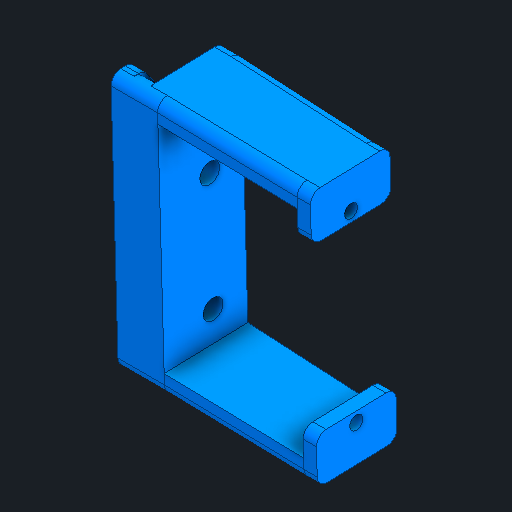
# Autodesk Inventor part: servo_mount
Saved by Autodesk Inventor 2023 (Build 270158030, 158C)
## iProperties
Created: 2022-03-29
Part Number: servo_mount
Material: Generic
Document SubType Name: Modeling
Designer: kardo
Density: 1 g/cm^3
Appearance: Blue Plastic
Author: kardo
Autodesk Inventor part; units mm, degrees
ref_plane "YZ Plane" through (0, 0, 0) normal (1, 0, 0) x (0, 1, 0)
ref_plane "XZ Plane" through (0, 0, 0) normal (0, 1, 0) x (-1, 0, 0)
ref_plane "XY Plane" through (0, 0, 0) normal (0, 0, 1) x (1, 0, 0)
derived "stencil_frame.ipt"
sketch "sk_servo_mount" plane through (-54.6, 0, 0) normal (1, 0, 0) x (0, 1, 0)
  line L0 (-254.1001, 21.0191) -> (9.48, 28.5282) construction
  line L1 (-363, 4666.1952) -> (-363, -2045.0469) construction
  line L2 (0, 4666.1952) -> (0, -2045.0469) construction
  line L3 (-204.8284, 22.4228) -> (-205.0163, 29.0201) construction
  line L4 (-205.0163, 29.0201) -> (-187.0237, 29.5327) construction
  line L5 (-187.0237, 29.5327) -> (-186.8357, 22.9354) construction
  point P0 (0, 0)
  point P1 (-196.02, 29.2764)
ref_plane "plane_cowl_left" through (-54.6, 0, 0) normal (1, 0, 0) x (0, 1, 0)
derived "parameters_frame.ipt"
derived "parameters_powertrain.ipt"
derived "parameters_hardware.ipt"
ref_plane "plane_inner_stringer" through (-54.6, -254.1001, 21.0191) normal (1, 0, 0) x (0, 0.9995944, 0.0284775)
ref_plane "plane_fastening" through (-28.6, -254.1001, 21.0191) normal (1, 0, 0) x (0, 0.9995944, 0.0284775)
ref_plane "plane_servo_rod_joint" through (-14.6, -254.1001, 21.0191) normal (1, 0, 0) x (0, 0.9995944, 0.0284775)
sketch "sk_fastening" plane through (-28.6, -254.1001, 21.0191) normal (1, 0, 0) x (0, 0.9995944, 0.0284775)
  line L0 (49.2917, 6.6) -> (67.2917, 6.6) construction
  line L1 (58.2917, 6.6) -> (58.2917, 106.6) construction
  line L2 (58.2917, 106.6) -> (158.2917, 106.6) construction
  line L3 (158.2917, 106.6) -> (158.2917, 22.6) construction
  line L4 (158.2917, 22.6) -> (66.2917, 22.6) construction
  line L5 (66.2917, 22.6) -> (66.2917, 8.6) construction
  line L6 (66.2917, 8.6) -> (61.2917, 8.6) construction
  line L7 (44.7917, 14.6) -> (44.7917, 2.6)
  line L8 (44.7917, 2.6) -> (48.7917, 2.6)
  line L9 (48.7917, 2.6) -> (48.7917, 14.6)
  line L10 (48.7917, 14.6) -> (44.7917, 14.6)
  line L11 (73.7917, 14.6) -> (73.7917, 2.6)
  line L12 (73.7917, 2.6) -> (77.7917, 2.6)
  line L13 (77.7917, 2.6) -> (77.7917, 14.6)
  line L14 (77.7917, 14.6) -> (73.7917, 14.6)
  line L15 (48.7917, 14.6) -> (73.7917, 14.6) construction
  line L16 (73.7917, 2.6) -> (48.7917, 2.6) construction
  line L17 (61.2917, 2.6) -> (61.2917, 14.6) construction
  line L18 (44.7917, 14.6) -> (41.7917, 14.6)
  line L19 (41.7917, 14.6) -> (41.7917, 2.6)
  line L20 (41.7917, 2.6) -> (44.7917, 2.6)
  line L21 (77.7917, 14.6) -> (80.7917, 14.6)
  line L22 (80.7917, 14.6) -> (80.7917, 2.6)
  line L23 (80.7917, 2.6) -> (77.7917, 2.6)
  line L24 (47.2917, 8.6) -> (48.7917, 8.6) construction
  line L25 (73.7917, 8.6) -> (75.2917, 8.6) construction
  point P0 (253.3985, -28.2467)
  point P1 (61.2917, 8.6)
  dimension "d46" = 100
  dimension "d47" = 84
  dimension "d49" = 100
  dimension "d50" = 92
  dimension "d52" = 14
  dimension "d53" = 5
  dimension "d54" = 25
  dimension "d55" = 33
  dimension "d56" = 3
  dimension "d57" = 3
  dimension "d58" = 12
  dimension "d59" = 28
  constraints: 50 end point, 8 collinear, 8 perpendicular, 7 parallel, 5 midpoint, 2 point on line, 1 coincident, 1 other
  measures "d46" distance of L1.end L2.end
  measures "d47" distance of L2.end L3.end
  measures "d49" distance of L1.start L1.end
  measures "d50" distance of L3.end L4.end
  measures "d52" distance of L4.end L5.end
  measures "d53" distance of L6.end L5.end
  measures "d54" distance between parallel lines of L11 L9
  measures "d55" distance between parallel lines of L13 L7
  measures "d56" distance of L7.start L18.end
  measures "d57" distance of L13.end L21.end
  measures "d58" distance of L21.end L22.end
  measures "d59" distance of L25.end L24.start
sketch "sk_base" plane through (-54.6, -254.1001, 21.0191) normal (1, 0, 0) x (0, 0.9995944, 0.0284775)
  line L0 (44.7917, 14.6) -> (41.7917, 14.6) construction
  line L1 (41.7917, 14.6) -> (41.7917, 2.6) construction
  line L2 (41.7917, 2.6) -> (44.7917, 2.6) construction
  line L3 (80.7917, 2.6) -> (77.7917, 2.6) construction
  line L4 (80.7917, 14.6) -> (80.7917, 2.6) construction
  line L5 (77.7917, 14.6) -> (80.7917, 14.6) construction
  line L6 (49.2917, 6.6) -> (67.2917, 6.6) construction
  line L7 (0, 0) -> (263.6871, 0) construction
  line L8 (41.7917, 1.5) -> (80.7917, 1.5)
  line L9 (80.7917, 1.5) -> (80.7917, 14.1)
  line L10 (80.7917, 14.1) -> (41.7917, 14.1)
  line L11 (41.7917, 14.1) -> (41.7917, 1.5)
  line L12 (49.2917, 6.6) -> (41.7917, 6.6) construction
  line L13 (49.2917, 6.6) -> (49.2917, 14.1) construction
  line L14 (67.2917, 6.6) -> (80.7917, 6.6) construction
  line L15 (67.2917, 6.6) -> (67.2917, 14.1) construction
  point P0 (253.3985, -28.2467)
  point P1 (61.2917, 8.6)
  point P2 (58.2917, 6.6)
  dimension "d60" = 22.5
  dimension "d61" = 16.5
  dimension "d62" = 18
  dimension "d64" = 1.5
  dimension "d65" = 7.5
  dimension "d66" = 16.5
  dimension "d67" = 22.5
  constraints: 16 end point, 6 perpendicular, 4 point on line, 2 parallel
  measures "d60" distance from line of L4 point (58.292, 6.6)
  measures "d61" distance from line of L1 point (58.292, 6.6)
  measures "d62" distance of L6.start L6.end
  measures "d64" distance between parallel lines of L7 L8
  measures "d65" distance of L12.start L13.end
  measures "d66" distance from line of point (58.292, 6.6) L11
  measures "d67" distance from line of point (58.292, 6.6) L9
ref_plane "plane_column_bottom" through (-52.1, -254.1001, 21.0191) normal (1, 0, 0) x (0, 0.9995944, 0.0284775)
ref_plane "plane_outer_plate" through (-57.1, -254.1001, 21.0191) normal (1, 0, 0) x (0, 0.9995944, 0.0284775)
sketch "sk_hex_holes" plane through (-57.1, -254.1001, 21.0191) normal (1, 0, 0) x (0, 0.9995944, 0.0284775)
  line L0 (50.8794, 9.35) -> (52.4671, 6.6)
  line L1 (52.4671, 6.6) -> (50.8794, 3.85)
  line L2 (50.8794, 3.85) -> (47.704, 3.85)
  line L3 (47.704, 3.85) -> (46.1163, 6.6)
  line L4 (46.1163, 6.6) -> (47.704, 9.35)
  line L5 (47.704, 9.35) -> (50.8794, 9.35)
  line L6 (68.8794, 9.35) -> (70.4671, 6.6)
  line L7 (70.4671, 6.6) -> (68.8794, 3.85)
  line L8 (68.8794, 3.85) -> (65.704, 3.85)
  line L9 (65.704, 3.85) -> (64.1163, 6.6)
  line L10 (64.1163, 6.6) -> (65.704, 9.35)
  line L11 (65.704, 9.35) -> (68.8794, 9.35)
  point P0 (253.3985, -28.2467)
  point P1 (49.2917, 6.6)
  point P2 (67.2917, 6.6)
  point P3 (49.2917, 6.6)
  point P4 (67.2917, 6.6)
  dimension "d102" = 5.5
  constraints: 24 end point, 2 coincident, 2 collinear, 26 other
  measures "d102" distance between parallel lines of L2 L5
sketch "sk_bridge" plane through (-54.6, -254.1001, 21.0191) normal (1, 0, 0) x (0, 0.9995944, 0.0284775)
  line L0 (80.7917, 14.1) -> (41.7917, 14.1) projected
  line L1 (41.7917, 14.1) -> (41.7917, 1.5) projected
  line L2 (80.7917, 1.5) -> (80.7917, 14.1) projected
  line L3 (41.7917, 11.1) -> (80.7917, 11.1)
  point P0 (253.3985, -28.2467)
  dimension "d70" = 3
  constraints: 2 end point, 2 point on line, 1 parallel
  measures "d70" distance between parallel lines of L0 L3
sketch "sk_backplate" plane through (-57.1, -254.1001, 21.0191) normal (1, 0, 0) x (0, 0.9995944, 0.0284775)
  line L0 (41.7917, 14.1) -> (41.7917, 1.5) construction
  line L1 (80.7917, 14.1) -> (41.7917, 14.1) projected
  line L2 (80.7917, 1.5) -> (80.7917, 14.1) construction
  line L3 (68.8794, 3.85) -> (65.704, 3.85) projected
  line L4 (50.8794, 3.85) -> (47.704, 3.85) projected
  line L5 (80.7917, 14.1) -> (80.7917, 11.1)
  line L6 (72.0548, 3.85) -> (68.8794, 3.85)
  line L7 (65.704, 3.85) -> (50.8794, 3.85)
  line L8 (47.704, 3.85) -> (44.5286, 3.85)
  line L9 (41.7917, 14.1) -> (41.7917, 11.1)
  line L10 (47.704, 3.85) -> (46.1163, 6.6) construction
  line L11 (41.7917, 11.1) -> (80.7917, 11.1) construction
  line L12 (70.4671, 6.6) -> (68.8794, 3.85) construction
  line L13 (44.5286, 3.85) -> (42.9408, 6.6)
  line L14 (42.9408, 6.6) -> (41.7917, 11.1)
  line L15 (80.7917, 11.1) -> (73.6426, 6.6)
  line L16 (73.6426, 6.6) -> (72.0548, 3.85)
  point P0 (253.3985, -28.2467)
  constraints: 18 end point, 4 equal length, 2 collinear, 2 parallel
ref_plane "plane_column_top" through (-30.6, -254.1001, 21.0191) normal (1, 0, 0) x (0, 0.9995944, 0.0284775)
extrude "extrude_fastening_plates" add sketch "sk_fastening" against normal up to surface (2 mm away)
extrude "extrude_backplate" add sketch "sk_backplate" against normal blind 2
extrude "extrude_front_plate" add sketch "sk_base" along normal up to surface (2.5 mm away)
extrude "extrude_bridge" add sketch "sk_bridge" against normal up to surface (2.5 mm away)
sketch "sk_column_bottom_1" plane through (-52.1, -254.1001, 21.0191) normal (1, 0, 0) x (0, 0.9995944, 0.0284775)
  line L0 (80.7917, 14.1) -> (41.7917, 14.1) construction
  line L1 (41.7917, 1.5) -> (80.7917, 1.5) construction
  line L2 (44.7917, 14.6) -> (44.7917, 2.6) construction
  line L3 (41.7917, 14.6) -> (41.7917, 2.6) construction
  line L4 (41.7917, 14.1) -> (44.7917, 14.1)
  line L5 (44.7917, 14.1) -> (44.7917, 1.5)
  line L6 (44.7917, 1.5) -> (41.7917, 1.5)
  line L7 (41.7917, 1.5) -> (41.7917, 14.1)
  point P0 (253.3985, -28.2467)
  constraints: 8 end point, 4 collinear
sketch "sk_column_top_1" plane through (-30.6, -254.1001, 21.0191) normal (1, 0, 0) x (0, 0.9995944, 0.0284775)
  line L0 (41.7917, 14.6) -> (41.7917, 2.6) projected
  line L1 (44.7917, 14.6) -> (41.7917, 14.6) projected
  line L2 (44.7917, 14.6) -> (44.7917, 2.6) projected
  line L3 (41.7917, 2.6) -> (44.7917, 2.6) projected
  point P0 (253.3985, -28.2467)
sketch "sk_column_bottom_2" plane through (-52.1, -254.1001, 21.0191) normal (1, 0, 0) x (0, 0.9995944, 0.0284775)
  line L0 (77.7917, 2.6) -> (77.7917, 14.6) construction
  line L1 (80.7917, 14.6) -> (80.7917, 2.6) construction
  line L2 (80.7917, 14.1) -> (41.7917, 14.1) construction
  line L3 (41.7917, 1.5) -> (80.7917, 1.5) construction
  line L4 (77.7917, 14.1) -> (77.7917, 1.5)
  line L5 (77.7917, 1.5) -> (80.7917, 1.5)
  line L6 (80.7917, 1.5) -> (80.7917, 14.1)
  line L7 (80.7917, 14.1) -> (77.7917, 14.1)
  point P0 (253.3985, -28.2467)
  constraints: 8 end point, 4 collinear
sketch "sk_column_top_2" plane through (-30.6, -254.1001, 21.0191) normal (1, 0, 0) x (0, 0.9995944, 0.0284775)
  line L0 (77.7917, 2.6) -> (77.7917, 14.6) projected
  line L1 (80.7917, 14.6) -> (80.7917, 2.6) projected
  line L2 (77.7917, 14.6) -> (80.7917, 14.6) projected
  line L3 (80.7917, 2.6) -> (77.7917, 2.6) projected
  point P0 (253.3985, -28.2467)
loft "column_1" add profiles "sk_column_bottom_1", "sk_column_top_1"
loft "column_2" add profiles "sk_column_bottom_2", "sk_column_top_2"
hole "fastening_holes" at (-28.6, -207.0725, 30.9623) at (-28.6, -179.0838, 31.7597) direction (-1, 0, 0) diameter 2 depth 2 tip angle 118
hole "stringer_holes" at (-54.6, -187.0237, 29.5327) at (-54.6, -205.0163, 29.0201) direction (1, 0, 0) diameter 3 depth 2.5 tip angle 118
extrude "hex_holes" cut sketch "sk_hex_holes" against normal through all
fillet "fillet_outer_corners" radius 1.5 16 edges at (-41.35, -212.734, 36.5534) (-41.35, -212.3837, 24.2584) (-29.6, -212.3994, 24.8081) (-53.35, -212.3681, 23.7086) (-29.6, -212.7411, 36.8033) (-29.6, -173.7569, 37.9139) (-41.35, -173.7498, 37.664) (-55.6, -173.7427, 37.4141) (-29.6, -173.4152, 25.9188) (-41.35, -173.3996, 25.369) (-53.35, -173.3839, 24.8192) (-29.6, -205.744, 37.0026) (-29.6, -205.4022, 25.0075) (-29.6, -180.7541, 37.7145) (-29.6, -180.4124, 25.7194) (-55.6, -212.7269, 36.3035)
fillet "fillet_backplate" radius 1.5 8 edges at (-58.1, -173.6573, 34.4153) (-55.85, -173.6573, 34.4153) (-58.1, -180.6754, 29.7135) (-58.1, -182.1841, 26.9194) (-58.1, -209.6992, 26.1356) (-58.1, -211.3646, 28.8392) (-58.1, -212.6415, 33.3047) (-55.85, -212.6415, 33.3047)
equation "\"d52\" = servo_arm_length"
equation "\"d53\" = servo_axis_location"
equation "\"d55\" = servo_length_fastening"
equation "\"d58\" = servo_width"
equation "\"d59\" = servo_fastening_distance"
equation "\"d88\" = servo_fastening_diam"
equation "\"d95\" = drill_servo_mount_diam"
equation "\"d44\" = servo_height_fastening - servo_height_joint"
equation "\"servo_arm_length\" = 14"
equation "\"servo_axis_location\" = 5"
equation "\"servo_length_fastening\" = 33"
equation "\"servo_width\" = 12"
equation "\"servo_fastening_distance\" = 28"
equation "\"servo_fastening_diam\" = 2"
equation "\"drill_servo_mount_diam\" = 3"
equation "\"servo_height_fastening\" = 20"
equation "\"servo_height_joint\" = 34"
body "Solid2"
